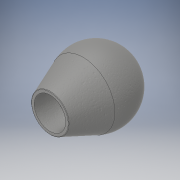
# Autodesk Inventor part: FilmLamp
Saved by Autodesk Inventor 2018.2 (Build 222227000, 227)
## iProperties
Created: 2018-01-26
Part Number: FilmLamp
Material: Beton
Document SubType Name: Modeling
Designer: JochenAlt
Density: 2.40731 g/cm^3
Appearance: Textur - grau
Author: JochenAlt
Autodesk Inventor part; units mm, degrees
ref_plane "YZ Plane" through (0, 0, 0) normal (1, 0, 0) x (0, 1, 0)
ref_plane "XZ Plane" through (0, 0, 0) normal (0, 1, 0) x (-1, 0, 0)
ref_plane "XY Plane" through (0, 0, 0) normal (0, 0, 1) x (1, 0, 0)
sketch "Skizze1" plane through (0, 0, 0) normal (0, 0, 1) x (1, 0, 0)
  line L0 (0, 102.5527) -> (0, -110.5912) construction
  line L1 (-15.2336, 0) -> (91.4016, 0) construction
  line L2 (6, 59.6992) -> (6, 49.6387)
  line L3 (24.3229, -43.6852) -> (27.5, -80)
  line L4 (31.8243, -80) -> (27.5, -80)
  arc A0 (55.6679, -22.3849) -> (6, 59.6992) centre (0, 0) ccw
  arc A1 (24.3229, -43.6852) -> (6, 49.6387) centre (0, 0) ccw
  line L5 (55.6679, -22.3849) -> (32.7521, -79.3731)
  arc A2 (31.8243, -80) -> (32.7521, -79.3731) centre (31.8243, -79) ccw
  point P0 (32.5, -80)
  dimension "d3" = 6
  dimension "d10" = 50
  dimension "d11" = 60
  dimension "d12" = 5
  dimension "d13" = 80
  dimension "d15" = 5
  dimension "d16" = 27.5
  dimension "d17" = 1
  constraints: 8 end point, 6 point on circle, 3 centre point, 3 tangent, 2 coincident, 2 point on line, 1 horizontal, 1 vertical
  measures "d3" distance between parallel lines of L2 L0
  measures "d10" radius of A1
  measures "d11" radius of A0
  measures "d12" angle of L0 L3
  measures "d13" distance between parallel lines of L1 L4
  measures "d15" distance of point (32.5, -80) L3.end
  measures "d16" distance from line of L0 L3.end
  measures "d17" radius of A2
revolve "Umdrehung1" add sketch "Skizze1" angle 360 about axis through (0, 0, 0) along (0, -1, 0)
